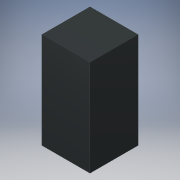
# Autodesk Inventor part: laser
Saved by Autodesk Inventor 2019 (Build 230136000, 136)
## iProperties
Created: 2019-03-11
Part Number: laser
Material: Iron, Cast
Document SubType Name: Modeling
Designer: Saumya
Density: 7.15 g/cm^3
Appearance: Iron Gray
Author: Saumya
Autodesk Inventor part; units mm, degrees
ref_plane "YZ Plane" through (0, 0, 0) normal (1, 0, 0) x (0, 1, 0)
ref_plane "XZ Plane" through (0, 0, 0) normal (0, 1, 0) x (-1, 0, 0)
ref_plane "XY Plane" through (0, 0, 0) normal (0, 0, 1) x (1, 0, 0)
sketch "Sketch1" plane through (0, 0, 0) normal (0, 0, 1) x (1, 0, 0)
  line L0 (63.5852, 104.9902) -> (114.3852, 104.9902)
  line L1 (114.3852, 104.9902) -> (114.3852, 3.3902)
  line L2 (114.3852, 3.3902) -> (63.5852, 3.3902)
  line L3 (63.5852, 3.3902) -> (63.5852, 104.9902)
  point P0 (0, 0)
  dimension "d0" = 50.8
  dimension "d1" = 101.6
  constraints: 8 end point, 2 parallel, 1 horizontal, 1 perpendicular
  measures "d0" distance of L0.start L0.end
  measures "d1" distance of L0.end L1.end
extrude "Extrusion1" add sketch "Sketch1" along normal blind 50.8
sketch "Sketch2" plane through (63.5852, 3.3902, 0) normal (0, -1, 0) x (1, 0, 0)
  circle A0 centre (25.8879, 25.992) radius 12.2628
  point P0 (-63.5852, 0)
  constraints: 1 centre point
extrude "Extrusion2" cut sketch "Sketch2" against normal blind 25.4
body "Solid1"
